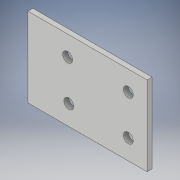
# Autodesk Inventor part: gusset 1
Saved by Autodesk Inventor 2017 (Build 210142000, 142)
## iProperties
Created: 2017-12-29
Part Number: gusset 1
Material: Generic
Document SubType Name: Modeling
Designer: Micah
Density: 1 g/cm^3
Appearance: Default
Author: Micah
Autodesk Inventor part; units mm, degrees
ref_plane "YZ Plane" through (0, 0, 0) normal (1, 0, 0) x (0, 1, 0)
ref_plane "XZ Plane" through (0, 0, 0) normal (0, 1, 0) x (-1, 0, 0)
ref_plane "XY Plane" through (0, 0, 0) normal (0, 0, 1) x (1, 0, 0)
sketch "Sketch1" plane through (0, 0, 0) normal (0, 0, 1) x (1, 0, 0)
  line L0 (0, 0) -> (76.2, 0)
  line L1 (76.2, 0) -> (76.2, 50.8)
  line L2 (76.2, 50.8) -> (0, 50.8)
  line L3 (0, 50.8) -> (0, 0)
  circle A0 centre (25.4, 38.1) radius 3.175
  circle A1 centre (26.1775, 12.7) radius 3.175
  circle A2 centre (64.1876, 38.1) radius 3.175
  circle A3 centre (64.1876, 12.7) radius 3.175
  dimension "d0" = 76.2
  dimension "d1" = 50.8
  dimension "d2" = 6.35
  dimension "d3" = 6.35
  dimension "d4" = 25.4
  dimension "d5" = 12.7
  dimension "d6" = 25.4
  dimension "d7" = 6.35
  dimension "d8" = 6.35
  dimension "d9" = 25.4
  dimension "d12" = 12.7
  constraints: 8 end point, 4 centre point, 2 parallel, 1 horizontal, 1 perpendicular
  measures "d0" distance of L2.end L1.end
  measures "d1" distance of L1.end L0.end
  measures "d2" diameter of A0
  measures "d3" diameter of A1
  measures "d4" vertical distance of A1.centre A0.centre
  measures "d5" distance from line of L2 A0.centre
  measures "d6" distance from line of A0.centre L3
  measures "d7" diameter of A2
  measures "d8" diameter of A3
  measures "d9" distance of A3.centre A2.centre
  measures "d12" distance from line of L2 A2.centre
extrude "Extrusion1" add sketch "Sketch1" along normal blind 3.175
body "Solid1"
